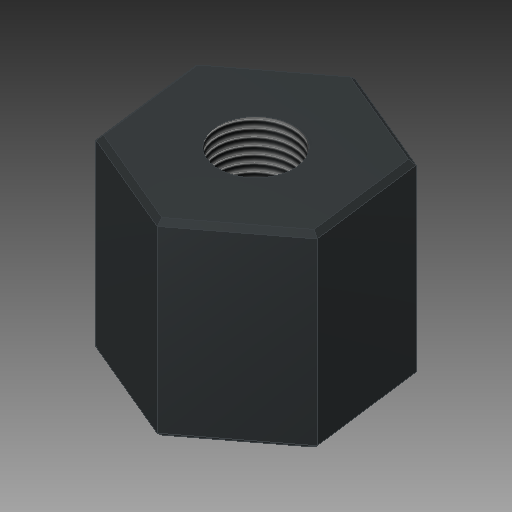
# Autodesk Inventor part: 5M nut 20mm
Saved by Autodesk Inventor 2018 (Build 220112000, 112)
## iProperties
Created: 2017-11-24
Part Number: 5M nut 20mm
Material: Iron, Gray
Document SubType Name: Modeling
Designer: g
Density: 7.15 g/cm^3
Appearance: Iron Gray
Author: g
Autodesk Inventor part; units mm, degrees
ref_plane "YZ Plane" through (0, 0, 0) normal (1, 0, 0) x (0, 1, 0)
ref_plane "XZ Plane" through (0, 0, 0) normal (0, 1, 0) x (-1, 0, 0)
ref_plane "XY Plane" through (0, 0, 0) normal (0, 0, 1) x (1, 0, 0)
sketch "Sketch1" plane through (0, 0, 0) normal (0, 1, 0) x (-1, 0, 0)
  circle A0 centre (0, 0) radius 4
  line L0 (11.1804, -4.6903) -> (1.5283, -12.0276)
  line L1 (1.5283, -12.0276) -> (-9.6521, -7.3374)
  line L2 (-9.6521, -7.3374) -> (-11.1804, 4.6903)
  line L3 (-11.1804, 4.6903) -> (-1.5283, 12.0276)
  line L4 (-1.5283, 12.0276) -> (9.6521, 7.3374)
  line L5 (9.6521, 7.3374) -> (11.1804, -4.6903)
  dimension "d0" = 8
  dimension "d19" = 10.5
  constraints: 12 end point, 2 coincident, 1 centre point, 13 other
  measures "d0" diameter of A0
  measures "d19" distance from line of point (0, 0) L5
extrude "Extrusion1" add sketch "Sketch1" along normal blind 20
thread "Thread1" size "M5x0.8" class "6H" standard "ANSI Metric M Profile" full length
chamfer "Chamfer1" distance 0.5 angle 45 12 edges at (-4.0619, 0, 9.6825) (6.3543, 0, 8.359) (10.4162, 0, -1.3235) (4.0619, 0, -9.6825) (-6.3543, 0, -8.359) (-10.4162, 0, 1.3235) (-4.0619, 20, 9.6825) (-10.4162, 20, 1.3235) (6.3543, 20, 8.359) (-6.3543, 20, -8.359) (4.0619, 20, -9.6825) (10.4162, 20, -1.3235)
body "Solid1"
